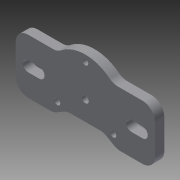
# Autodesk Inventor part: MountPlate
Saved by Autodesk Inventor 2014 SP1 (Build 180222100, 222)
## iProperties
Created: 2013-12-26
Part Number: MountPlate
Material: Generic
Document SubType Name: Modeling
Designer: Jack
Density: 1 g/cm^3
Appearance: Default
Author: Jack
Autodesk Inventor part; units mm, degrees
ref_plane "YZ Plane" through (0, 0, 0) normal (1, 0, 0) x (0, 1, 0)
ref_plane "XZ Plane" through (0, 0, 0) normal (0, 1, 0) x (-1, 0, 0)
ref_plane "XY Plane" through (0, 0, 0) normal (0, 0, 1) x (1, 0, 0)
sketch "Sketch1" plane through (0, 0, 0) normal (0, 1, 0) x (-1, 0, 0)
  line L0 (0, 0) -> (0, 27.94)
  line L1 (71.12, 27.94) -> (71.12, 0)
  arc A0 (49.5914, 27.94) -> (21.5286, 27.94) centre (35.56, 13.97) ccw
  line L2 (0, 27.94) -> (21.5286, 27.94)
  line L3 (49.5914, 27.94) -> (71.12, 27.94)
  circle A1 centre (35.56, 13.97) radius 16.5 construction
  circle A2 centre (35.56, 30.47) radius 1.5
  line L4 (35.56, 13.97) -> (49.8494, 5.72) construction
  line L5 (35.56, 13.97) -> (21.2706, 5.72) construction
  circle A3 centre (21.2706, 5.72) radius 1.5
  circle A4 centre (49.8494, 5.72) radius 1.5
  line L6 (71.12, 13.97) -> (0, 13.97) construction
  line L7 (51.7567, 0) -> (44.8805, 3.97)
  line L8 (19.3633, 0) -> (26.2395, 3.97)
  line L9 (44.8805, 3.97) -> (26.2395, 3.97)
  line L10 (59.055, 13.97) -> (64.775, 13.97) construction
  line L11 (59.055, 11.305) -> (64.775, 11.305)
  line L12 (64.775, 16.635) -> (59.055, 16.635)
  arc A5 (59.055, 16.635) -> (59.055, 11.305) centre (59.055, 13.97) ccw
  arc A6 (64.775, 11.305) -> (64.775, 16.635) centre (64.775, 13.97) ccw
  line L13 (6.33, 13.97) -> (12.08, 13.97) construction
  line L14 (6.33, 11.305) -> (12.08, 11.305)
  line L15 (12.08, 16.635) -> (6.33, 16.635)
  arc A7 (6.33, 16.635) -> (6.33, 11.305) centre (6.33, 13.97) ccw
  arc A8 (12.08, 11.305) -> (12.08, 16.635) centre (12.08, 13.97) ccw
  line L16 (71.12, 0) -> (51.7567, 0)
  line L17 (19.3633, 0) -> (0, 0)
  point P0 (61.915, 13.97)
  point P1 (9.205, 13.97)
  dimension "d0" = 27.94
  dimension "d1" = 71.12
  dimension "d5" = 35.56
  dimension "d7" = 19.8
  dimension "d8" = 33
  dimension "d9" = 3
  dimension "d10" = 3
  dimension "d11" = 3
  dimension "d13" = 30
  dimension "d14" = 4
  dimension "d15" = 4
  dimension "d16" = 10
  dimension "d17" = 2.86
  dimension "d18" = 5.33
  dimension "d19" = 2.875
  dimension "d20" = 5.33
  dimension "d21" = 26.355
  dimension "d22" = 26.355
  dimension "d23" = 13.97
  constraints: 40 end point, 13 point on circle, 10 parallel, 9 centre point, 8 tangent, 4 coincident, 4 midpoint, 4 point on line, 3 horizontal alignment, 2 perpendicular, 1 vertical, 1 vertical alignment
  measures "d0" distance of L0.start L0.end
  measures "d1" distance of L0.end L1.start
  measures "d5" distance from line of L1 point (35.56, 13.97)
  measures "d7" radius of A0
  measures "d8" diameter of A1
  measures "d9" diameter of A2
  measures "d10" diameter of A3
  measures "d11" diameter of A4
  measures "d13" angle of L6 L4
  measures "d14" distance from line of L4.end L7
  measures "d15" distance from line of L5.end L8
  measures "d16" distance from line of L4.start L9
  measures "d17" distance of point (61.915, 13.97) L10.end
  measures "d18" diameter of A6
  measures "d19" distance of point (9.205, 13.97) L13.end
  measures "d20" diameter of A8
  measures "d21" distance of A0.centre point (9.205, 13.97)
  measures "d22" distance of L4.start point (61.915, 13.97)
  measures "d23" distance from line of L17 A0.centre
extrude "Extrusion1" add sketch "Sketch1" along normal blind 4.763
fillet "Fillet1" radius 6.35 10 edges at (0, 2.3815, 0) (0, 2.3815, 27.94) (-71.12, 2.3815, 0) (-71.12, 2.3815, 27.94) (-21.5286, 2.3815, 27.94) (-49.5914, 2.3815, 27.94) (-26.2395, 2.3815, 3.97) (-19.3633, 2.3815, 0) (-44.8805, 2.3815, 3.97) (-51.7567, 2.3815, 0)
sketch "Sketch2" plane through (0, 4.763, 0) normal (0, 1, 0) x (1, 0, 0)
  arc A0 (-48.0228, -29.3557) -> (-23.0972, -29.3557) centre (-35.56, -13.97) ccw projected
  circle A1 centre (-35.56, -13.97) radius 3.4
  point P0 (0, 0)
  dimension "d27" = 6.8
  constraints: 1 centre point, 1 coincident
  measures "d27" diameter of A1
extrude "Extrusion2" cut sketch "Sketch2" against normal blind 3
sketch "Sketch3" plane through (-35.56, 1.763, 13.97) normal (0, 1, 0) x (1, 0, 0)
  circle A0 centre (0, 0) radius 3.4 projected
  circle A1 centre (0, 0) radius 1.75
  point P0 (35.56, 13.97)
  dimension "d30" = 3.5
  constraints: 1 centre point, 1 coincident
  measures "d30" diameter of A1
extrude "Extrusion3" cut sketch "Sketch3" against normal blind 6.75 contours A1
body "Solid1"
